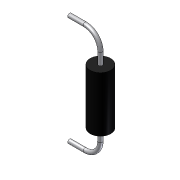
# Autodesk Inventor part: VISHAY-DALE RWR81S6R98FRB12
Saved by Autodesk Inventor 2014 SP1 (Build 180222100, 222)
## iProperties
Created: 2012-11-10
Part Number: VISHAY-DALE RWR81S6R98FRB12
Document SubType Name: Modeling
Designer: Robert Davis
Density: 2.11 g/cm^3
Material: SMT (95% LCP, 5% PhosBr)
Mass: 0.0898806 g
Surface Area: 0.922059 cm^2
Volume: 0.0425975 cm^3
Description: WIREWOUND RESISTOR, 6.98 OHM
Appearance: Default
Author: Robert Davis
Autodesk Inventor part; units mm, degrees
ref_plane "YZ Plane" through (0, 0, 0) normal (1, 0, 0) x (0, 1, 0)
ref_plane "XZ Plane" through (0, 0, 0) normal (0, 1, 0) x (-1, 0, 0)
ref_plane "XY Plane" through (0, 0, 0) normal (0, 0, 1) x (1, 0, 0)
sketch "Sketch1" plane through (0, 0, 0) normal (0, 0, 1) x (1, 0, 0)
  circle A0 centre (0, 0) radius 1.3341
  dimension "d0" = 2.6682
  constraints: 1 centre point
  measures "d0" diameter of A0
extrude "Extrusion1" add sketch "Sketch1" along normal mid plane 7.137
sketch "Sketch2" plane through (0, 0, 3.5685) normal (0, 0, 1) x (1, 0, 0)
  circle A0 centre (0, 0) radius 0.25
  dimension "d7" = 0.5
  constraints: 1 centre point
  measures "d7" diameter of A0
sketch3d "3D Sketch2"
  constraints: 2 horizontal
sweep "Sweep1" [suppressed]
sketch "Sketch3" plane through (0, 0, -3.5685) normal (0, 0, -1) x (-1, 0, 0)
  circle A0 centre (0, 0) radius 0.25
  dimension "d18" = 0.5
  constraints: 1 centre point
  measures "d18" diameter of A0
sketch3d "3D Sketch3"
  constraints: 2 vertical
sweep "Sweep2" [suppressed]
sketch "Sketch4" plane through (0, 0, 3.5685) normal (0, 0, 1) x (1, 0, 0)
  circle A0 centre (0, 0) radius 0.25
  dimension "d25" = 0.5
  constraints: 1 centre point
  measures "d25" diameter of A0
sketch3d "3D Sketch4"
  constraints: 2 vertical
sweep "Sweep3" [suppressed]
sketch "Sketch5" plane through (0, 0, -3.5685) normal (0, 0, -1) x (-1, 0, 0)
  circle A0 centre (0, 0) radius 0.254
  dimension "d34" = 0.508
  constraints: 1 centre point
  measures "d34" diameter of A0
sketch3d "3D Sketch5"
  line L0 (0, 0, -3.5685) -> (0, 0, -5.0685)
  arc A0 (0, 0, -5.0685) -> (-2, 0, -7.0685) centre (-2, 0, -5.0685) ccw
  line L1 (-2, 0, -7.0685) -> (-4, 0, -7.0685)
  dimension "d52" = 3.5
  dimension "d53" = 4
  dimension "d36" = 2
  constraints: 2 vertical
sweep "Sweep4" add profiles "Sketch5" path "3D Sketch5"
sketch "Sketch7" plane through (0, 0, 3.5685) normal (0, 0, 1) x (1, 0, 0)
  circle A0 centre (0, 0) radius 1.3341 projected
  circle A1 centre (0, 0) radius 0.254
  dimension "d45" = 0.508
  constraints: 1 centre point
  measures "d45" diameter of A1
sketch3d "3D Sketch7"
  constraints: 2 vertical
sweep "Sweep6" [suppressed]
mirror "Mirror2" about plane through (0, 0, 0) normal (0, 0, 1) of "Sweep4"
body "Solid1"
